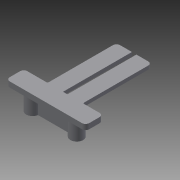
# Autodesk Inventor part: Top Tube Holder
Saved by Autodesk Inventor 2015 (Build 190159000, 159)
## iProperties
Created: 2016-05-27
Part Number: Top Tube Holder
Material: Generic
Document SubType Name: Modeling
Designer: Toby
Density: 1 g/cm^3
Appearance: Default
Author: Toby
Autodesk Inventor part; units mm, degrees
ref_plane "YZ Plane" through (0, 0, 0) normal (1, 0, 0) x (0, 1, 0)
ref_plane "XZ Plane" through (0, 0, 0) normal (0, 1, 0) x (-1, 0, 0)
ref_plane "XY Plane" through (0, 0, 0) normal (0, 0, 1) x (1, 0, 0)
sketch "Sketch1" plane through (0, 0, 0) normal (0, 0, 1) x (1, 0, 0)
  line L0 (-35.6553, 6.44) -> (9.3447, 6.44)
  line L1 (9.3447, 6.44) -> (9.3447, -3.56)
  line L2 (9.3447, -3.56) -> (-35.6553, -3.56)
  line L3 (-35.6553, -3.56) -> (-35.6553, 6.44)
  line L4 (-23.1553, 6.44) -> (-3.1553, 6.44)
  line L5 (-3.1553, 6.44) -> (-3.1553, 46.44)
  line L6 (-3.1553, 46.44) -> (-23.1553, 46.44)
  line L7 (-23.1553, 46.44) -> (-23.1553, 6.44)
  point P0 (0, 0)
  dimension "d0" = 20
  dimension "d1" = 10
  dimension "d2" = 40
  dimension "d3" = 12.5
  dimension "d4" = 12.5
  dimension "d5" = 45
  constraints: 16 end point, 4 parallel, 2 horizontal, 2 perpendicular, 1 point on line
  measures "d0" distance of L5.end L6.end
  measures "d1" distance of L2.end L0.start
  measures "d2" distance of L6.end L4.start
  measures "d3" distance between parallel lines of L3 L7
  measures "d4" distance between parallel lines of L1 L5
  measures "d5" distance of L1.end L2.end
extrude "Extrusion1" add sketch "Sketch1" along normal blind 2
sketch "Sketch2" plane through (0, 0, 2) normal (0, 0, 1) x (1, 0, 0)
  circle A0 centre (-25.6553, 1.44) radius 2.6
  circle A1 centre (-0.6553, 1.44) radius 2.6
  line L0 (9.3447, -3.56) -> (9.3447, 6.44) projected
  line L1 (-35.6553, -3.56) -> (9.3447, -3.56) projected
  point P0 (0, 0)
  dimension "d8" = 5.2
  dimension "d9" = 10
  dimension "d10" = 25
  dimension "d11" = 5.2
  dimension "d12" = 5
  dimension "d13" = 5
  constraints: 2 centre point
  measures "d8" diameter of A0
  measures "d9" distance from line of L0 A1.centre
  measures "d10" distance of A0.centre A1.centre
  measures "d11" diameter of A1
  measures "d12" distance from line of L1 A0.centre
  measures "d13" distance from line of L1 A1.centre
extrude "Extrusion2" cut sketch "Sketch2" against normal blind 2
sketch "Sketch3" plane through (0, 0, 2) normal (0, 0, 1) x (1, 0, 0)
  line L0 (-35.6553, -3.56) -> (9.3447, -3.56)
  line L1 (9.3447, -3.56) -> (9.3447, 6.44)
  line L2 (9.3447, 6.44) -> (-35.6553, 6.44)
  line L3 (-35.6553, 6.44) -> (-35.6553, -3.56)
  point P0 (0, 0)
  constraints: 8 end point, 2 parallel, 1 horizontal, 1 perpendicular
extrude "Extrusion3" add sketch "Sketch3" along normal blind 1
sketch "Sketch4" plane through (0, 0, 2) normal (0, 0, 1) x (1, 0, 0)
  line L0 (-23.1553, 6.44) -> (-3.1553, 6.44) projected
  line L1 (-14.4053, 6.44) -> (-11.9053, 6.44)
  line L2 (-11.9053, 6.44) -> (-11.9053, 46.44)
  line L3 (-11.9053, 46.44) -> (-14.4053, 46.44)
  line L4 (-14.4053, 46.44) -> (-14.4053, 6.44)
  line L5 (-23.1553, 46.44) -> (-23.1553, 6.44) projected
  line L6 (-3.1553, 6.44) -> (-3.1553, 46.44) projected
  point P0 (0, 0)
  dimension "d18" = 2.5
  dimension "d19" = 40
  dimension "d20" = 8.75
  dimension "d21" = 8.75
  constraints: 8 end point, 2 parallel, 1 horizontal, 1 perpendicular, 1 point on line
  measures "d18" distance between parallel lines of L2 L4
  measures "d19" distance of L3.end L1.start
  measures "d20" distance between parallel lines of L5 L4
  measures "d21" distance between parallel lines of L6 L2
extrude "Extrusion4" cut sketch "Sketch4" against normal blind 2
fillet "Fillet1" radius 2 6 edges at (-35.6553, 6.44, 1.5) (9.3447, 6.44, 1.5) (-3.1553, 46.44, 1) (-23.1553, 46.44, 1) (-3.1553, 6.44, 1) (-23.1553, 6.44, 1)
fillet "Fillet2" radius 2 2 edges at (9.3447, -3.56, 1.5) (-35.6553, -3.56, 1.5)
sketch "Sketch5" plane through (0, 0, 0) normal (0, 0, -1) x (-1, 0, 0)
  circle A0 centre (0.6553, 1.44) radius 2.6 projected
  circle A1 centre (0.6553, 1.44) radius 2.6
  circle A2 centre (25.6553, 1.44) radius 2.6 projected
  circle A3 centre (25.6553, 1.44) radius 2.6
  circle A4 centre (25.6553, 1.44) radius 3.6
  circle A5 centre (0.6553, 1.44) radius 3.6
  point P0 (0, 0)
  dimension "d26" = 7.2
  dimension "d27" = 7.2
  constraints: 4 centre point, 4 coincident
  measures "d26" diameter of A5
  measures "d27" diameter of A4
extrude "Extrusion5" add sketch "Sketch5" along normal blind 10
sketch "Sketch6" plane through (0, 0, 0) normal (0, 0, -1) x (-1, 0, 0)
  line L0 (3.6821, 0.94) -> (22.6767, 0.94)
  line L1 (22.6767, 0.94) -> (22.6767, 1.94)
  line L2 (22.6767, 1.94) -> (3.6821, 1.94)
  line L3 (3.6821, 1.94) -> (3.6821, 0.94)
  circle A0 centre (0.6553, 1.44) radius 2.6 projected
  point P0 (0, 0)
  dimension "d30" = 0.5
  dimension "d31" = 0.5
  constraints: 8 end point, 2 parallel, 1 horizontal, 1 perpendicular
  measures "d30" distance from line of A0.centre L0
  measures "d31" distance from line of A0.centre L2
extrude "Extrusion6" add sketch "Sketch6" along normal blind 10 contours L3 L2 L1 L0
body "Solid1"
